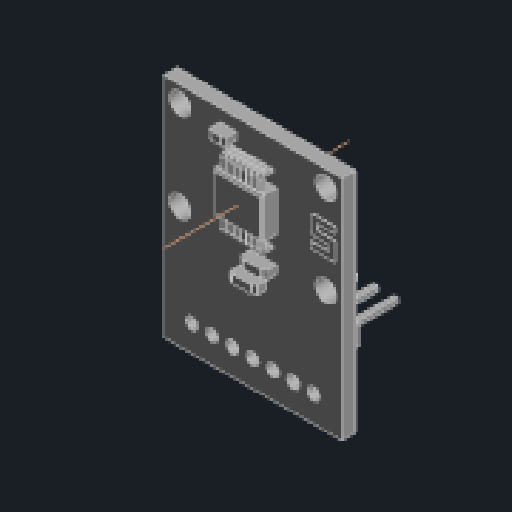
# Autodesk Inventor part: AS5040-AB-2.2-DemoBoard
Saved by Autodesk Inventor 2025.2 (Build 292293000, 293)
## iProperties
Created: 2025-11-07
Part Number: AS5040-AB-2.2-DemoBoard
Material: Generic
Document SubType Name: Modeling
Designer: valer
Density: 1 g/cm^3
Appearance: Default
Author: valer
Autodesk Inventor part; units mm, degrees
ref_plane "YZ Plane" through (0, 0, 0) normal (1, 0, 0) x (0, 1, 0)
ref_plane "XZ Plane" through (0, 0, 0) normal (0, 1, 0) x (-1, 0, 0)
ref_plane "XY Plane" through (0, 0, 0) normal (0, 0, 1) x (1, 0, 0)
sketch "Base" plane through (0, 0, 0) normal (0, 0, 1) x (1, 0, 0)
  line L0 (-11, -14) -> (11, -14)
  line L1 (11, -14) -> (11, 14)
  line L2 (11, 14) -> (-11, 14)
  line L3 (-11, 14) -> (-11, -14)
  line L4 (-11, -14) -> (11, 14) construction
  line L5 (11, -14) -> (-11, 14) construction
  circle A0 centre (-9, 12) radius 1.3
  line L6 (0, -19.6) -> (0, 19.6) construction
  line L7 (-10.3, 10.7) -> (-7.7, 10.7) construction
  line L8 (-7.7, 10.7) -> (-7.7, 13.3) construction
  line L9 (-7.7, 13.3) -> (-10.3, 13.3) construction
  line L10 (-10.3, 13.3) -> (-10.3, 10.7) construction
  line L11 (-10.3, 10.7) -> (-7.7, 13.3) construction
  line L12 (-7.7, 10.7) -> (-10.3, 13.3) construction
  circle A1 centre (9, 12) radius 1.3
  line L13 (-11, 6.5) -> (11, 6.5) construction
  circle A2 centre (-9, 1) radius 1.3
  circle A3 centre (9, 1) radius 1.3
  line L14 (-9, 1) -> (9, 12) construction
  line L15 (9, -12) -> (-9, -12)
  line L16 (-9, -12) -> (-9, -9.5)
  line L17 (-9, -9.5) -> (9, -9.5)
  line L18 (9, -9.5) -> (9, -12)
  line L19 (9, -7) -> (-9, -7)
  line L20 (-9, -7) -> (-9, -4.5)
  line L21 (-9, -4.5) -> (9, -4.5)
  line L22 (9, -4.5) -> (9, -7)
  line L23 (9, -10.75) -> (-9, -10.75) construction
  circle A4 centre (7.5, -10.75) radius 0.75
  circle A5 centre (5, -10.75) radius 0.75
  circle A6 centre (2.5, -10.75) radius 0.75
  circle A7 centre (0, -10.75) radius 0.75
  circle A8 centre (-2.5, -10.75) radius 0.75
  circle A9 centre (-5, -10.75) radius 0.75
  circle A10 centre (-7.5, -10.75) radius 0.75
  line L24 (9, -9.5) -> (9, -7) construction
  line L25 (-9, -9.5) -> (-9, -7) construction
  line L26 (9, -8.25) -> (-9, -8.25) construction
  circle A11 centre (7.5, -5.75) radius 0.75
  circle A12 centre (5, -5.75) radius 0.75
  circle A13 centre (2.5, -5.75) radius 0.75
  circle A14 centre (0, -5.75) radius 0.75
  circle A15 centre (-2.5, -5.75) radius 0.75
  circle A16 centre (-5, -5.75) radius 0.75
  circle A17 centre (-7.5, -5.75) radius 0.75
  line L27 (3, 9) -> (-3, 9)
  line L28 (-3, 9) -> (-3, 4)
  line L29 (-3, 4) -> (3, 4)
  line L30 (3, 4) -> (3, 9)
  line L31 (3, 9) -> (-3, 4) construction
  line L32 (-3, 9) -> (3, 4) construction
  point P0 (0, 0)
  point P1 (0, 6.5)
  dimension "d0" = 22
  dimension "d1" = 28
  dimension "d2" = 2.6
  dimension "d4" = 0.7
  dimension "d5" = 0.7
  dimension "d6" = 18
  dimension "d7" = 11
  dimension "d8" = 2.5
  dimension "d9" = 2
  dimension "d10" = 2.5
  dimension "d11" = 2
  dimension "d12" = 2
  dimension "d13" = 1.5
  dimension "d16" = 2.5
  dimension "d21" = 1.5
  dimension "d22" = 1.5
  dimension "d23" = 6
  dimension "d24" = 5
  constraints: 64 end point, 18 centre point, 11 midpoint, 10 parallel, 10 symmetric about line, 6 horizontal, 6 perpendicular, 5 point on line, 2 tangent, 2 vertical, 1 collinear, 22 other
  measures "d0" distance of L1.end L2.end
  measures "d1" distance of L0.end L1.end
  measures "d2" diameter of A0
  measures "d4" distance between parallel lines of L3 L10
  measures "d5" distance between parallel lines of L2 L9
  measures "d6" distance of L14.end A0.centre
  measures "d7" distance of L14.start A0.centre
  measures "d8" distance of L17.end L15.start
  measures "d9" distance between parallel lines of L0 L15
  measures "d10" distance between parallel lines of L19 L17
  measures "d11" distance between parallel lines of L1 L18
  measures "d12" distance between parallel lines of L3 L16
  measures "d13" distance from line of A4.centre L18
  measures "d16" distance of A4.centre A5.centre
  measures "d21" distance from line of L16 A10.centre
  measures "d22" diameter of A4
  measures "d23" distance of L27.start L27.end
  measures "d24" distance between parallel lines of L27 L29
extrude "BaseFeature" add sketch "Base" against normal blind 1.7 contours L3 L2 L1 L0 | L15 L16 L17 L18 | L19 L20 L21 L22 | A4 | A5 | A6 | A7 | A8 | A9 | A10 | A11 | A12 | A13 | A14 | A15 | A16 | A17 | L30 L29 L28 L27
extrude "ICFeature" add sketch "Base" along normal blind 1.9 contours L30 L29 L28 L27
chamfer "ICChamferFeature" distance 0.25 angle 45 4 edges at (0, 4, 1.9) (-3, 6.5, 1.9) (0, 9, 1.9) (3, 6.5, 1.9)
extrude "PinsBaseFeature" add sketch "Base" against normal blind 4.2 contours L19 L20 L21 L22 | A11 | A12 | A13 | A14 | A15 | A16 | A17
sketch "Sketch2" plane through (0, 0, -4.2) normal (0, 0, -1) x (-1, 0, 0)
  circle A0 centre (-7.5, -10.75) radius 0.75 projected
  circle A1 centre (-5, -10.75) radius 0.75 projected
  circle A2 centre (-2.5, -10.75) radius 0.75 projected
  circle A3 centre (0, -10.75) radius 0.75 projected
  circle A4 centre (2.5, -10.75) radius 0.75 projected
  circle A5 centre (5, -10.75) radius 0.75 projected
  circle A6 centre (7.5, -10.75) radius 0.75 projected
  circle A7 centre (-7.5, -5.75) radius 0.75 projected
  circle A8 centre (-5, -5.75) radius 0.75 projected
  circle A9 centre (-2.5, -5.75) radius 0.75 projected
  circle A10 centre (0, -5.75) radius 0.75 projected
  circle A11 centre (2.5, -5.75) radius 0.75 projected
  circle A12 centre (5, -5.75) radius 0.75 projected
  circle A13 centre (7.5, -5.75) radius 0.75 projected
  line L0 (7.8, -10.45) -> (7.2, -10.45)
  line L1 (7.2, -10.45) -> (7.2, -11.05)
  line L2 (7.2, -11.05) -> (7.8, -11.05)
  line L3 (7.8, -11.05) -> (7.8, -10.45)
  line L4 (7.8, -10.45) -> (7.2, -11.05) construction
  line L5 (7.2, -10.45) -> (7.8, -11.05) construction
  line L6 (5.3, -10.45) -> (4.7, -10.45)
  line L7 (4.7, -10.45) -> (4.7, -11.05)
  line L8 (4.7, -11.05) -> (5.3, -11.05)
  line L9 (5.3, -11.05) -> (5.3, -10.45)
  line L10 (5.3, -10.45) -> (4.7, -11.05) construction
  line L11 (4.7, -10.45) -> (5.3, -11.05) construction
  line L12 (2.8, -10.45) -> (2.2, -10.45)
  line L13 (2.2, -10.45) -> (2.2, -11.05)
  line L14 (2.2, -11.05) -> (2.8, -11.05)
  line L15 (2.8, -11.05) -> (2.8, -10.45)
  line L16 (2.8, -10.45) -> (2.2, -11.05) construction
  line L17 (2.2, -10.45) -> (2.8, -11.05) construction
  line L18 (0.3, -10.45) -> (-0.3, -10.45)
  line L19 (-0.3, -10.45) -> (-0.3, -11.05)
  line L20 (-0.3, -11.05) -> (0.3, -11.05)
  line L21 (0.3, -11.05) -> (0.3, -10.45)
  line L22 (0.3, -10.45) -> (-0.3, -11.05) construction
  line L23 (-0.3, -10.45) -> (0.3, -11.05) construction
  line L24 (-2.2, -10.45) -> (-2.8, -10.45)
  line L25 (-2.8, -10.45) -> (-2.8, -11.05)
  line L26 (-2.8, -11.05) -> (-2.2, -11.05)
  line L27 (-2.2, -11.05) -> (-2.2, -10.45)
  line L28 (-2.2, -10.45) -> (-2.8, -11.05) construction
  line L29 (-2.8, -10.45) -> (-2.2, -11.05) construction
  line L30 (-4.7, -10.45) -> (-5.3, -10.45)
  line L31 (-5.3, -10.45) -> (-5.3, -11.05)
  line L32 (-5.3, -11.05) -> (-4.7, -11.05)
  line L33 (-4.7, -11.05) -> (-4.7, -10.45)
  line L34 (-4.7, -10.45) -> (-5.3, -11.05) construction
  line L35 (-5.3, -10.45) -> (-4.7, -11.05) construction
  line L36 (-7.2, -10.45) -> (-7.8, -10.45)
  line L37 (-7.8, -10.45) -> (-7.8, -11.05)
  line L38 (-7.8, -11.05) -> (-7.2, -11.05)
  line L39 (-7.2, -11.05) -> (-7.2, -10.45)
  line L40 (-7.2, -10.45) -> (-7.8, -11.05) construction
  line L41 (-7.8, -10.45) -> (-7.2, -11.05) construction
  line L42 (7.8, -5.45) -> (7.2, -5.45)
  line L43 (7.2, -5.45) -> (7.2, -6.05)
  line L44 (7.2, -6.05) -> (7.8, -6.05)
  line L45 (7.8, -6.05) -> (7.8, -5.45)
  line L46 (7.8, -5.45) -> (7.2, -6.05) construction
  line L47 (7.2, -5.45) -> (7.8, -6.05) construction
  line L48 (5.3, -5.45) -> (4.7, -5.45)
  line L49 (4.7, -5.45) -> (4.7, -6.05)
  line L50 (4.7, -6.05) -> (5.3, -6.05)
  line L51 (5.3, -6.05) -> (5.3, -5.45)
  line L52 (5.3, -5.45) -> (4.7, -6.05) construction
  line L53 (4.7, -5.45) -> (5.3, -6.05) construction
  line L54 (2.8, -5.45) -> (2.2, -5.45)
  line L55 (2.2, -5.45) -> (2.2, -6.05)
  line L56 (2.2, -6.05) -> (2.8, -6.05)
  line L57 (2.8, -6.05) -> (2.8, -5.45)
  line L58 (2.8, -5.45) -> (2.2, -6.05) construction
  line L59 (2.2, -5.45) -> (2.8, -6.05) construction
  line L60 (0.3, -5.45) -> (-0.3, -5.45)
  line L61 (-0.3, -5.45) -> (-0.3, -6.05)
  line L62 (-0.3, -6.05) -> (0.3, -6.05)
  line L63 (0.3, -6.05) -> (0.3, -5.45)
  line L64 (0.3, -5.45) -> (-0.3, -6.05) construction
  line L65 (-0.3, -5.45) -> (0.3, -6.05) construction
  line L66 (-2.2, -5.45) -> (-2.8, -5.45)
  line L67 (-2.8, -5.45) -> (-2.8, -6.05)
  line L68 (-2.8, -6.05) -> (-2.2, -6.05)
  line L69 (-2.2, -6.05) -> (-2.2, -5.45)
  line L70 (-2.2, -5.45) -> (-2.8, -6.05) construction
  line L71 (-2.8, -5.45) -> (-2.2, -6.05) construction
  line L72 (-4.7, -5.45) -> (-5.3, -5.45)
  line L73 (-5.3, -5.45) -> (-5.3, -6.05)
  line L74 (-5.3, -6.05) -> (-4.7, -6.05)
  line L75 (-4.7, -6.05) -> (-4.7, -5.45)
  line L76 (-4.7, -5.45) -> (-5.3, -6.05) construction
  line L77 (-5.3, -5.45) -> (-4.7, -6.05) construction
  line L78 (-7.2, -5.45) -> (-7.8, -5.45)
  line L79 (-7.8, -5.45) -> (-7.8, -6.05)
  line L80 (-7.8, -6.05) -> (-7.2, -6.05)
  line L81 (-7.2, -6.05) -> (-7.2, -5.45)
  line L82 (-7.2, -5.45) -> (-7.8, -6.05) construction
  line L83 (-7.8, -5.45) -> (-7.2, -6.05) construction
  point P0 (0, 0)
  dimension "d34" = 0.6
  constraints: 168 end point, 28 midpoint, 28 parallel, 20 equal length, 14 horizontal, 14 perpendicular, 7 point on line
  measures "d34" distance of L2.end L1.end
extrude "PinsFeature" add sketch "Sketch2" along normal blind 6 contours L45 L44 L43 L42 | L51 L50 L49 L48 | L57 L56 L55 L54 | L63 L62 L61 L60 | L69 L68 L67 L66 | L75 L74 L73 L72 | L81 L80 L79 L78
extrude "ThroughHolesFeature" cut sketch "Base" against normal through all contours A4 | A5 | A6 | A7 | A8 | A9 | A10
sketch "BoardParts" plane through (0, 0, 0) normal (0, 0, 1) x (1, 0, 0)
  line L0 (3, 4) -> (-3, 4) projected
  line L1 (2.5, 4) -> (2, 4)
  line L2 (2, 4) -> (2, 2.2)
  line L3 (2, 2.2) -> (2.5, 2.2)
  line L4 (2.5, 2.2) -> (2.5, 4)
  line L5 (3, 4) -> (3, 9) projected
  line L6 (1.86, 2.2) -> (1.86, 4)
  line L7 (1.36, 2.2) -> (1.86, 2.2)
  line L8 (1.36, 4) -> (1.36, 2.2)
  line L9 (1.86, 4) -> (1.36, 4)
  line L10 (1.22, 2.2) -> (1.22, 4)
  line L11 (0.72, 2.2) -> (1.22, 2.2)
  line L12 (0.72, 4) -> (0.72, 2.2)
  line L13 (1.22, 4) -> (0.72, 4)
  line L14 (0.58, 2.2) -> (0.58, 4)
  line L15 (0.08, 2.2) -> (0.58, 2.2)
  line L16 (0.08, 4) -> (0.08, 2.2)
  line L17 (0.58, 4) -> (0.08, 4)
  line L18 (-0.06, 2.2) -> (-0.06, 4)
  line L19 (-0.56, 2.2) -> (-0.06, 2.2)
  line L20 (-0.56, 4) -> (-0.56, 2.2)
  line L21 (-0.06, 4) -> (-0.56, 4)
  line L22 (-0.7, 2.2) -> (-0.7, 4)
  line L23 (-1.2, 2.2) -> (-0.7, 2.2)
  line L24 (-1.2, 4) -> (-1.2, 2.2)
  line L25 (-0.7, 4) -> (-1.2, 4)
  line L26 (-1.34, 2.2) -> (-1.34, 4)
  line L27 (-1.84, 2.2) -> (-1.34, 2.2)
  line L28 (-1.84, 4) -> (-1.84, 2.2)
  line L29 (-1.34, 4) -> (-1.84, 4)
  line L30 (-1.98, 2.2) -> (-1.98, 4)
  line L31 (-2.48, 2.2) -> (-1.98, 2.2)
  line L32 (-2.48, 4) -> (-2.48, 2.2)
  line L33 (-1.98, 4) -> (-2.48, 4)
  line L34 (3, 9) -> (3, 4) projected
  line L35 (3, 6.5) -> (-3, 6.5) construction
  line L36 (-3, 4) -> (-3, 9) projected
  line L37 (1.75, -2.5) -> (-1.5, -2.5)
  line L38 (-1.5, -2.5) -> (-1.5, -1.5)
  line L39 (-1.5, -1.5) -> (1.75, -1.5)
  line L40 (1.75, -1.5) -> (1.75, -2.5)
  line L41 (11, -14) -> (11, 14) projected
  line L42 (-11, -14) -> (11, -14) projected
  line L43 (3, -0.25) -> (-0.25, -0.25)
  line L44 (-0.25, -0.25) -> (-0.25, 0.75)
  line L45 (-0.25, 0.75) -> (3, 0.75)
  line L46 (3, 0.75) -> (3, -0.25)
  line L47 (2, 9) -> (2, 10.8)
  line L48 (2, 10.8) -> (2.5, 10.8)
  line L49 (2.5, 10.8) -> (2.5, 9)
  line L50 (1.86, 10.8) -> (1.86, 9)
  line L51 (1.36, 10.8) -> (1.86, 10.8)
  line L52 (1.36, 9) -> (1.36, 10.8)
  line L53 (1.22, 10.8) -> (1.22, 9)
  line L54 (0.72, 10.8) -> (1.22, 10.8)
  line L55 (0.72, 9) -> (0.72, 10.8)
  line L56 (0.58, 10.8) -> (0.58, 9)
  line L57 (0.08, 10.8) -> (0.58, 10.8)
  line L58 (0.08, 9) -> (0.08, 10.8)
  line L59 (-0.06, 10.8) -> (-0.06, 9)
  line L60 (-0.56, 10.8) -> (-0.06, 10.8)
  line L61 (-0.56, 9) -> (-0.56, 10.8)
  line L62 (-0.7, 10.8) -> (-0.7, 9)
  line L63 (-1.2, 10.8) -> (-0.7, 10.8)
  line L64 (-1.2, 9) -> (-1.2, 10.8)
  line L65 (-1.34, 10.8) -> (-1.34, 9)
  line L66 (-1.84, 10.8) -> (-1.34, 10.8)
  line L67 (-1.84, 9) -> (-1.84, 10.8)
  line L68 (-1.98, 10.8) -> (-1.98, 9)
  line L69 (-2.48, 10.8) -> (-1.98, 10.8)
  line L70 (-2.48, 9) -> (-2.48, 10.8)
  line L71 (-3, 9) -> (3, 9) projected
  point P0 (0, 0)
  point P1 (1.75, -2)
  point P2 (3, 0.25)
  dimension "d39" = 0.5
  dimension "d40" = 0.5
  dimension "d43" = 0.64
  dimension "d48" = 1
  dimension "d49" = 3.25
  dimension "d50" = 9.25
  dimension "d51" = 11.5
  dimension "d52" = 1.25
  dimension "d53" = 8
  dimension "d56" = 1.8
  constraints: 130 end point, 32 symmetric about line, 8 parallel, 4 horizontal, 4 midpoint, 3 perpendicular, 1 point on line, 57 other
  measures "d39" distance between parallel lines of L2 L4
  measures "d40" distance between parallel lines of L5 L4
  measures "d43" distance of L3.end L6.start
  measures "d48" distance between parallel lines of L39 L37
  measures "d49" distance of L37.start L37.end
  measures "d50" distance from line of L41 point (1.75, -2)
  measures "d51" distance between parallel lines of L42 L37
  measures "d52" distance between parallel lines of L39 L43
  measures "d53" distance from line of L41 point (3, 0.25)
  measures "d56" distance of L32.start L31.start
extrude "LegsFeature" add sketch "BoardParts" along normal blind 1.5 contours L4 L3 L2 L0 | L71 L47 L48 L49 | L6 L7 L8 L0 | L71 L52 L51 L50 | L10 L11 L12 L0 | L71 L55 L54 L53 | L14 L15 L16 L0 | L71 L58 L57 L56 | L18 L19 L20 L0 | L71 L61 L60 L59 | L22 L23 L24 L0 | L71 L64 L63 L62 | L26 L27 L28 L0 | L71 L67 L66 L65 | L30 L31 L32 L0 | L71 L70 L69 L68
fillet "LegFilletsFeature" radius 0.5 16 edges at (-2.23, 2.2, 1.5) (-1.59, 2.2, 1.5) (-0.95, 2.2, 1.5) (-0.31, 2.2, 1.5) (0.33, 2.2, 1.5) (0.97, 2.2, 1.5) (1.61, 2.2, 1.5) (2.25, 2.2, 1.5) (2.25, 10.8, 1.5) (1.61, 10.8, 1.5) (0.97, 10.8, 1.5) (0.33, 10.8, 1.5) (-0.31, 10.8, 1.5) (-0.95, 10.8, 1.5) (-1.59, 10.8, 1.5) (-2.23, 10.8, 1.5)
sketch "Sketch4" plane through (2.5, 2.2, 0) normal (1, 0, 0) x (0, 0, -1)
  arc A0 (-1.5, 0.5) -> (-1, 0) centre (-1, 0.5) ccw projected
  line L0 (0, 0) -> (-1, 0) projected
  line L1 (0, 1.8) -> (0, 0) projected
  line L2 (-1.5, 1.8) -> (0, 1.8) projected
  line L3 (-1.5, 0.5) -> (-1.5, 1.8) projected
  arc A1 (-1, 8.6) -> (-1.5, 8.1) centre (-1, 8.1) ccw projected
  line L4 (-1.5, 6.8) -> (-1.5, 8.1) projected
  line L5 (0, 6.8) -> (-1.5, 6.8) projected
  line L6 (0, 8.6) -> (0, 6.8) projected
  line L7 (0, 8.6) -> (-1, 8.6) projected
  line L8 (-1.1, 1.4) -> (-0.4, 1.4)
  line L9 (-0.4, 1.4) -> (-0.4, 0.4) construction
  line L10 (-0.4, 0.4) -> (-1, 0.4)
  arc A2 (-1.1, 0.5) -> (-1, 0.4) centre (-1, 0.5) ccw
  line L11 (-1.1, 0.5) -> (-1.1, 1.4)
  arc A3 (-1, 8.2) -> (-1.1, 8.1) centre (-1, 8.1) ccw
  line L12 (-1, 8.2) -> (-0.4, 8.2)
  line L13 (-0.4, 8.2) -> (-0.4, 7.2) construction
  line L14 (-0.4, 7.2) -> (-1.1, 7.2)
  line L15 (-1.1, 7.2) -> (-1.1, 8.1)
  line L16 (-0.4, 0.4) -> (0, 0.4)
  line L17 (-0.4, 1.4) -> (0, 1.4)
  line L18 (-0.4, 7.2) -> (0, 7.2)
  line L19 (-0.4, 8.2) -> (0, 8.2)
  line L20 (-1.1, 1.4) -> (-1.1, 1.8)
  line L21 (-1.1, 7.2) -> (-1.1, 6.8)
  point P0 (0, -2.2)
  dimension "d58" = 0.4
  dimension "d59" = 0.4
  constraints: 28 end point, 7 point on line, 5 perpendicular, 4 point on circle, 2 centre point, 8 other
  measures "d58" distance between parallel lines of L3 L11
  measures "d59" distance between parallel lines of L4 L15
extrude "LegInsideFeature" cut sketch "Sketch4" against normal through all contours L2 L1 L17 L8 L20 | L16 L10 A2 L11 L8 L17 L1 | L6 L18 L14 L15 A3 L12 L19 | L21 L14 L18 L6 L5
extrude "CapacitorsFeature" add sketch "BoardParts" along normal blind 1.5 contours L37 L38 L39 L40 | L43 L44 L45 L46
sketch "Sketch5" plane through (0, 0, 1.5) normal (0, 0, 1) x (1, 0, 0)
  line L0 (1.75, -1.5) -> (-1.5, -1.5) projected
  line L1 (-1.5, -1.5) -> (-1.5, -2.5) projected
  line L2 (-1.5, -2.5) -> (1.75, -2.5) projected
  line L3 (1.75, -2.5) -> (1.75, -1.5) projected
  line L4 (3, 0.75) -> (-0.25, 0.75) projected
  line L5 (-0.25, 0.75) -> (-0.25, -0.25) projected
  line L6 (-0.25, -0.25) -> (3, -0.25) projected
  line L7 (3, -0.25) -> (3, 0.75) projected
  line L8 (-1.5, -2.5) -> (1.75, -2.5) projected
  line L9 (-1, -2.5) -> (-1, -1.5)
  line L10 (1.25, -2.5) -> (1.25, -1.5)
  line L11 (-0.25, -0.25) -> (3, -0.25) projected
  line L12 (0.25, -0.25) -> (0.25, 0.75)
  line L13 (2.5, -0.25) -> (2.5, 0.75)
  line L14 (3, 0.75) -> (-0.25, 0.75) projected
  line L15 (1.75, -2.5) -> (1.75, -1.5) projected
  point P0 (0, 0)
  dimension "d64" = 0.5
  dimension "d65" = 0.5
  dimension "d66" = 0.5
  dimension "d67" = 0.5
  constraints: 8 end point, 8 point on line, 5 perpendicular, 1 parallel
  measures "d64" distance between parallel lines of L1 L9
  measures "d65" distance between parallel lines of L3 L10
  measures "d66" distance between parallel lines of L5 L12
  measures "d67" distance between parallel lines of L7 L13
extrude "CapacitorDetailFeature" cut sketch "Sketch5" against normal blind 0.25 contours L3 L2 L10 L0 | L9 L2 L1 L0 | L7 L6 L13 L4 | L12 L6 L5 L4
sketch "ResistorAndLogo" plane through (0, 0, 0) normal (0, 0, 1) x (1, 0, 0)
  line L0 (-2, 11.5) -> (-4, 11.5)
  line L1 (-4, 11.5) -> (-4, 12.5)
  line L2 (-4, 12.5) -> (-2, 12.5)
  line L3 (-2, 12.5) -> (-2, 11.5)
  line L4 (10.2389, 4.6725) -> (10.2389, 6.9558)
  line L5 (10.2389, 6.9558) -> (7.9556, 6.9558)
  line L6 (7.9556, 6.9558) -> (7.9556, 7.7169)
  line L7 (7.9556, 7.7169) -> (10.2389, 7.7169)
  line L8 (10.2389, 7.7169) -> (10.2389, 8.478)
  line L9 (10.2389, 8.478) -> (7.5751, 8.478)
  line L10 (7.5751, 8.478) -> (7.1945, 8.0975)
  line L11 (7.1945, 8.0975) -> (7.1945, 6.5753)
  line L12 (7.1945, 6.5753) -> (7.5751, 6.1947)
  line L13 (7.5751, 6.1947) -> (9.4778, 6.1947)
  line L14 (9.4778, 6.1947) -> (9.4778, 5.4336)
  line L15 (9.4778, 5.4336) -> (7.1945, 5.4336)
  line L16 (7.1945, 5.4336) -> (7.1945, 4.6725)
  line L17 (7.1945, 4.6725) -> (10.2389, 4.6725)
  line L18 (11, 14) -> (-11, 14) projected
  line L19 (-11, 14) -> (-11, -14) projected
  line L20 (11, -14) -> (11, 14) projected
  point P0 (0, 0)
  point P1 (9.4778, 5.8142)
  dimension "d70" = 1
  dimension "d71" = 1.5
  dimension "d72" = 7
  dimension "d73" = 2
  dimension "d74" = 0.7611
  dimension "d75" = 0.7611
  dimension "d76" = 0.7611
  dimension "d77" = 0.7611
  dimension "d78" = 3.0444
  dimension "d79" = 0.3805
  dimension "d80" = 0.3805
  dimension "d81" = 0.3805
  dimension "d83" = 0.7611
  dimension "d84" = 5.522
  dimension "d85" = 0.7611
  dimension "d86" = 0.7611
  dimension "d87" = 0.7611
  constraints: 36 end point, 9 perpendicular, 4 parallel, 4 point on line, 1 horizontal, 1 midpoint, 1 vertical
  measures "d70" distance between parallel lines of L2 L0
  measures "d71" distance between parallel lines of L18 L2
  measures "d72" distance from line of L19 L0.end
  measures "d73" distance of L1.end L2.end
  measures "d74" distance between parallel lines of L20 L4
  measures "d75" distance between parallel lines of L7 L5
  measures "d76" distance of L7.end L8.end
  measures "d77" distance of L15.end L16.end
  measures "d78" distance of L16.end L4.start
  measures "d79" distance from line of L11 L12.end
  measures "d80" horizontal distance of L10.end L9.end
  measures "d81" horizontal distance of L10.end L9.end
  measures "d83" distance between parallel lines of L13 L15
  measures "d84" distance between parallel lines of L18 L9
  measures "d85" distance between parallel lines of L5 L13
  measures "d86" distance between parallel lines of L11 L6
  measures "d87" distance from line of L4 point (9.478, 5.814)
extrude "ResistorFeature" add sketch "ResistorAndLogo" along normal blind 1.5 contours L0 L1 L2 L3
extrude "LogoFeature" add sketch "ResistorAndLogo" along normal blind 0.1 contours L17 L16 L15 L14 L13 L12 L11 L10 L9 L8 L7 L6 L5 L4
sketch "Sketch7" plane through (0, 0, 1.5) normal (0, 0, 1) x (1, 0, 0)
  line L0 (-2, 12.5) -> (-4, 12.5) projected
  line L1 (-4, 12.5) -> (-4, 11.5) projected
  line L2 (-4, 11.5) -> (-2, 11.5) projected
  line L3 (-2, 11.5) -> (-2, 12.5) projected
  line L4 (-4, 11.5) -> (-2, 11.5) projected
  line L5 (-3.5, 11.5) -> (-3.5, 12.5)
  line L6 (-2.5, 11.5) -> (-2.5, 12.5)
  line L7 (-4, 12.5) -> (-4, 11.5) projected
  point P0 (0, 0)
  point P1 (-4, 12)
  dimension "d92" = 0.5
  dimension "d93" = 0.5
  constraints: 4 end point, 4 point on line, 2 perpendicular, 1 midpoint
  measures "d92" distance from line of point (-4, 12) L5
  measures "d93" distance between parallel lines of L3 L6
extrude "Extrusion12" cut sketch "Sketch7" against normal blind 0.1 contours L3 L2 L6 L0 | L5 L2 L1 L0
equation "\"d5\" = d4"
equation "\"d11\" = d9"
equation "\"d12\" = d9"
equation "\"d21\" = d13"
equation "\"d74\" = d76"
equation "\"d75\" = d76"
equation "\"d77\" = d76"
equation "\"d78\" = 4 * d76"
equation "\"d79\" = 0.5 * d76"
equation "\"d80\" = d79"
equation "\"d81\" = d79"
equation "\"d83\" = d76"
equation "\"d85\" = d76"
equation "\"d86\" = d76"
equation "\"d87\" = d76"
body "Solid1"
